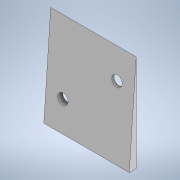
# Autodesk Inventor part: skos_smietnik1
Saved by Autodesk Inventor 2021 (Build 250183000, 183)
## iProperties
Created: 2025-11-29
Part Number: skos_smietnik1
Material: Generic
Document SubType Name: Modeling
Designer: huber
Density: 1 g/cm^3
Appearance: Default
Author: huber
Autodesk Inventor part; units mm, degrees
ref_plane "YZ Plane" through (0, 0, 0) normal (1, 0, 0) x (0, 1, 0)
ref_plane "XZ Plane" through (0, 0, 0) normal (0, 1, 0) x (-1, 0, 0)
ref_plane "XY Plane" through (0, 0, 0) normal (0, 0, 1) x (1, 0, 0)
sketch "Sketch1" plane through (0, 0, 0) normal (1, 0, 0) x (0, 1, 0)
  line L0 (0, 0) -> (74.6232, 0)
  line L1 (0, 0) -> (85, -6.078)
  line L2 (85, -6.078) -> (0, -6.078)
  line L3 (0, -6.078) -> (0, 0)
  dimension "d0" = 4.09
  dimension "d1" = 85
  constraints: 8 end point, 2 horizontal, 1 perpendicular
  measures "d0" angle of L2 L1
  measures "d1" distance from line of L1.end L3
extrude "Extrusion1" add sketch "Sketch1" along normal blind 75
sketch "Sketch2" plane through (0, 0, -6.078) normal (0, 0, -1) x (-1, 0, 0)
  line L0 (0, 0) -> (0, 85) projected
  line L1 (0, 85) -> (-75, 85) projected
  line L2 (-75, 0) -> (-75, 85) projected
  line L3 (0, 0) -> (-75, 0) projected
  point P0 (0, 0)
  point P1 (-15, 25)
  point P2 (-60, 60)
  dimension "d4" = 25
  dimension "d5" = 15
  dimension "d6" = 15
  dimension "d7" = 25
  measures "d4" distance from line of L3 point (-15, 25)
  measures "d5" distance from line of L0 point (-15, 25)
  measures "d6" distance from line of L2 point (-60, 60)
  measures "d7" distance from line of L1 point (-60, 60)
hole "Hole1" at (15, 25, -6.078) at (60, 60, -6.078) direction (0, 0, 1) diameter 9 depth 10 tip angle 118 clearance for "Socket Head Cap Screw ISO 4762" size "M8" standard "ISO"
body "Solid1"
